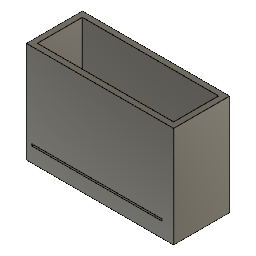
Storage box v3 (Autodesk Fusion 360 design; units mm, degrees)
Autodesk Fusion 360 part; units mm, degrees
box "BoxPrimitive1" add length 100 width 262.4458 height 180 placed x (0, 1, 0) y (-1, 0, 0) z (0, 0, 1) at (262.4458, 0, 0)
shell "Shell1" thickness 10 removed faces 1 at (87.4819, 33.3333, 180)
sketch "axle" plane through (10, 0, 0) normal (1, 0, 0) x (0, 1, 0)
  line L0 (90, 10) -> (90, 180)
  line L1 (90, 180) -> (10, 180)
  line L2 (10, 180) -> (10, 10)
  line L3 (10, 10) -> (90, 10)
  line L4 (10, 100) -> (90, 100) construction
  line L5 (50, 180) -> (50, 10) construction
  circle A0 centre (50, 100) radius 5
  dimension "d7" = 10
  constraint coincident L2 L4.start
  constraint coincident L0 L4.end
  constraint perpendicular L0 L4
  constraint midpoint L1 L5.start
  constraint midpoint L3 L5.end
  constraint coincident L5 A0.centre
  measures "d7" diameter of A0
extrude "Extrude1" add sketch "axle" along normal blind 240 contours A0
sketch "slot" plane through (0, 0, 0) normal (0, -1, 0) x (1, 0, 0)
  line L0 (0, 180) -> (0, 0)
  line L1 (0, 0) -> (262.4458, 0)
  line L2 (262.4458, 0) -> (262.4458, 180)
  line L3 (262.4458, 180) -> (0, 180)
  line L4 (10, 30) -> (241.775, 30)
  line L5 (241.775, 30) -> (241.775, 26.75)
  line L6 (241.775, 26.75) -> (10, 26.75)
  line L7 (10, 26.75) -> (10, 30)
  dimension "d10" = 231.775
  dimension "d11" = 3.25
  dimension "d12" = 10
  dimension "d13" = 26.75
  constraint horizontal L4
  constraint vertical L5
  constraint horizontal L6
  constraint vertical L7
  measures "d10" distance of L4.start L4.end
  measures "d11" distance of L4.end L5.end
  measures "d12" distance of L0 L6.end
  measures "d13" distance of L1 L6
extrude "Extrude2" cut sketch "slot" against normal blind 20 contours L4 L5 L6 L7
named bodies: "storage box"
